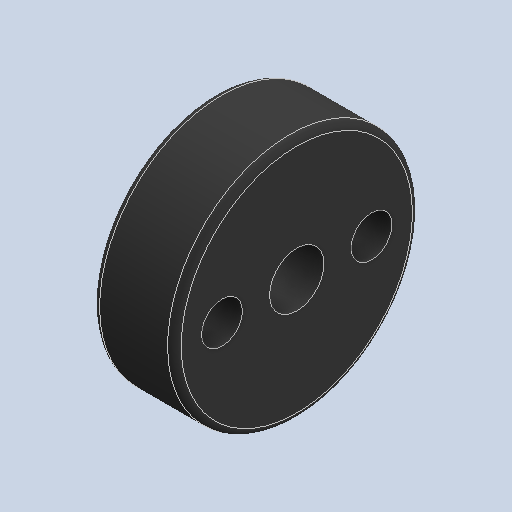
# Autodesk Inventor part: SCSWJ4-6_b
Saved by Autodesk Inventor 2025.1 (Build 291241000, 241)
## iProperties
Created: 2024-10-06
Part Number: SCSWJ4-6_b
Material: アルミニウム 6061
Document SubType Name: Modeling
Designer: haruy
Density: 2.7 g/cm^3
Appearance: ゴム - 黒
Author: haruy
Autodesk Inventor part; units mm, degrees
ref_plane "YZ Plane" through (0, 0, 0) normal (1, 0, 0) x (0, 1, 0)
ref_plane "XZ Plane" through (0, 0, 0) normal (0, 1, 0) x (-1, 0, 0)
ref_plane "XY Plane" through (0, 0, 0) normal (0, 0, 1) x (1, 0, 0)
sketch "スケッチ1" plane through (0, 0, 0) normal (1, 0, 0) x (0, 1, 0)
  circle A0 centre (0, 0) radius 9
  circle A1 centre (0, 0) radius 2
  circle A2 centre (0, 0) radius 5.5
  circle A3 centre (0, 5.5) radius 1.5
  circle A4 centre (0, -5.5) radius 1.5
  dimension "d0" = 18
  dimension "d1" = 4
  dimension "d2" = 11
  dimension "d3" = 3
  dimension "d4" = 3
  constraints: 5 centre point, 3 coincident, 2 point on circle
  measures "d0" diameter of A0
  measures "d1" diameter of A1
  measures "d2" diameter of A2
  measures "d3" diameter of A3
  measures "d4" diameter of A4
extrude "押し出し1" add sketch "スケッチ1" along normal blind 6 contours A0 | A2 A4 A3
fillet "フィレット1" radius 0.5 2 edges at (6, -9, 0) (0, -9, 0)
